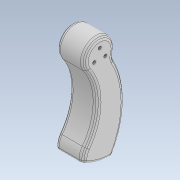
# Autodesk Inventor part: shank_link
Saved by Autodesk Inventor 2020 (Build 240168000, 168)
## iProperties
Created: 2020-12-22
Part Number: shank_link
Material: Generic
Document SubType Name: Modeling
Designer: DELL
Density: 1 g/cm^3
Appearance: Default
Author: DELL
Autodesk Inventor part; units mm, degrees
ref_plane "XZ Plane" through (0, 0, 0) normal (0, 1, 0) x (-1, 0, 0)
ref_plane "XY Plane" through (0, 0, 0) normal (0, 0, 1) x (1, 0, 0)
sketch "Sketch1" plane through (0, 0, 0) normal (1, 0, 0) x (0, 1, 0)
  line L0 (0, 0) -> (0, 36) construction
  line L1 (0, 0) -> (0, -36) construction
  line L2 (0, 0) -> (-150, 0) construction
  circle A0 centre (0, 0) radius 27.5
  arc A1 (-132.197115, 24.146579) -> (-15.713644, 22.568372) centre (-72.854167, 104.635178) ccw
  arc A2 (-9.117643, -25.944529) -> (-18.88547, -26.754596) centre (-13.096251, -37.265778) ccw
  arc A3 (-164.687324, -26.158794) -> (-18.88547, -26.754596) centre (-91.250706, 104.635178) ccw
  circle A4 centre (-150, 0) radius 30
  line L3 (-82.385192, -18.117333) -> (-150, 0) construction
  arc A5 (-152.527742, 29.893319) -> (-167.135748, -24.624503) centre (-82.385192, -18.117333) ccw
  circle A6 centre (0, 0) radius 11.5 construction
  circle A7 centre (11.5, 0) radius 1.65
  circle A8 centre (-5.75, 9.959292) radius 1.65
  circle A9 centre (-5.75, -9.959292) radius 1.65
  line L4 (0, 0) -> (-5.75, 9.959292) construction
  line L5 (0, 0) -> (-5.75, -9.959292) construction
  line L6 (0, 11.5) -> (0, -11.5) construction
  circle A10 centre (0, 0) radius 9.715 construction
  circle A11 centre (-9.715, 0) radius 2
  circle A12 centre (4.8575, 8.413437) radius 2
  circle A13 centre (4.8575, -8.413437) radius 2
  line L7 (0, 0) -> (5.75, 9.959292) construction
  line L8 (0, 0) -> (5.75, -9.959292) construction
  circle A14 centre (11.5, 0) radius 2.75
  circle A15 centre (-5.75, 9.959292) radius 2.75
  circle A16 centre (-5.75, -9.959292) radius 2.75
  point P0 (-75, 0)
  point P1 (13.433342, 23.995735)
  point P2 (-134.661731, -25.782504)
  point P3 (-13.946784, -23.700996)
  point P4 (-27.930718, 27.930718)
  point P5 (-134.537885, 25.708423)
  dimension "d83" = 23
  dimension "d5" = 55
  dimension "d16" = 150
  dimension "d22" = 200
  dimension "d28" = 150
  dimension "d75" = 60
  dimension "d76" = 70
  dimension "d80" = 15
  dimension "d81" = 85
  dimension "d82" = 12
  dimension "d84" = 3.3
  dimension "d85" = 30
  dimension "d86" = 30
  dimension "d87" = 19.43
  dimension "d88" = 4
  dimension "d89" = 30
  dimension "d90" = 5.5
  constraints: 19 point on circle, 18 end point, 16 centre point, 10 coincident, 6 equal radius, 5 tangent, 4 point on line, 3 midpoint, 2 horizontal alignment, 2 vertical, 1 perpendicular, 1 symmetric about line, 9 other
  measures "d5" diameter of A0
  measures "d16" distance of L0.start L2.end
  measures "d22" diameter of A1
  measures "d28" radius of A3
  measures "d75" diameter of A4
  measures "d76" distance of L3.start L3.end
  measures "d80" angle of L2 L3
  measures "d81" radius of A5
  measures "d82" radius of A2
  measures "d84" diameter of A7
  measures "d85" angle of L6 L4
  measures "d86" angle of L6 L5
  measures "d87" diameter of A10
  measures "d88" diameter of A12
  measures "d89" angle of L6 L7
  measures "d90" diameter of A14
ref_plane "Work Plane1" through (14.5, 0, 0) normal (1, 0, 0) x (0, 1, 0)
ref_plane "Work Plane2" through (-14.5, 0, 0) normal (1, 0, 0) x (0, 1, 0)
extrude "Extrusion4" add sketch "Sketch1" along normal mid plane 50 contours A0 | A0 A2 A3 A4 A1 | A4 A5 | A11 | A12 | A13 | A14 | A15 | A16 picked at (-149.80041, 0.261417)
extrude "Extrusion5" cut sketch "Sketch1" against normal blind 40 from surface at 25 contours A14 | A15 | A16
extrude "Extrusion6" cut sketch "Sketch1" along normal blind 10 from surface at -25 contours A11 | A12 | A13
chamfer "Chamfer5" distance 5 angle 45 10 edges at (25, -91.8637, -45.3636) (25, -14.088, -25.3068) (-25, -91.8637, -45.3636) (-25, -14.088, -25.3068) (25, -74.2089, 4.6444) (25, -141.8398, 28.8689) (25, -165.93, -25.4211) (-25, -74.2089, 4.6444) (-25, -165.93, -25.4211) (-25, -141.8398, 28.8689)
fillet "Fillet12" radius 5 32 edges at (0, -167.1357, -24.6245) (-25, -164.4889, 3.8823) (0, -152.5277, 29.8933) (25, -164.4889, 3.8823) (25, 22.2949, 3.0313) (25, -14.5013, -20.3239) (25, -91.8432, -40.3636) (25, -164.9357, -20.048) (25, -145.1567, 24.5264) (25, -74.2767, -0.3552) (20, -141.8398, 28.8689) (20, 27.2493, 3.7049) (20, -14.088, -25.3068) (20, -91.8637, -45.3636) (20, -165.93, -25.4211) (20, -74.2089, 4.6444) (-20, 27.2493, 3.7049) (-20, -14.088, -25.3068) (-20, -91.8637, -45.3636) (-20, -165.93, -25.4211) (-20, -141.8398, 28.8689) (-20, -74.2089, 4.6444) (-25, -145.1567, 24.5264) (-25, 22.2949, 3.0313) (-25, -14.5013, -20.3239) (-25, -91.8432, -40.3636) (-25, -164.9357, -20.048) (-25, -74.2767, -0.3552) (22.514, -167.3241, -21.3391) (22.514, -154.3336, 27.1422) (-22.514, -154.3336, 27.1422) (-22.514, -167.3241, -21.3391)
equation "\"d16\" = shank_length"
equation "\"shank_length\" = 150"
body "Solid1"
